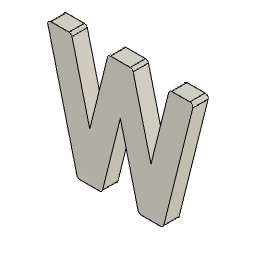
West (Autodesk Fusion 360 design; units mm, degrees)
Autodesk Fusion 360 part; units mm, degrees
sketch "Sketch1" plane through (0, 0, 0) normal (0, 1, 0) x (1, 0, 0)
  line L0 (1.6266, -50.8) -> (9.1684, -50.8)
  line L1 (0.3945, -49.222) -> (12.4595, -0.962)
  line L2 (13.6916, 0) -> (21.8684, 0)
  line L3 (26.3916, -50.8) -> (34.5684, -50.8)
  line L4 (30.48, -30.48) -> (23.1005, -0.962)
  line L5 (30.48, -30.48) -> (37.8595, -0.962)
  line L6 (39.0916, 0) -> (47.2684, 0)
  line L7 (43.18, -20.32) -> (35.8005, -49.838)
  line L8 (43.18, -20.32) -> (50.5595, -49.838)
  line L9 (51.7916, -50.8) -> (59.3334, -50.8)
  line L10 (60.5655, -49.222) -> (48.5005, -0.962)
  arc A0 (0.3945, -49.222) -> (1.6266, -50.8) centre (1.6266, -49.53) ccw
  arc A1 (9.1684, -50.8) -> (10.4005, -49.838) centre (9.1684, -49.53) ccw
  arc A2 (13.6916, 0) -> (12.4595, -0.962) centre (13.6916, -1.27) ccw
  arc A3 (23.1005, -0.962) -> (21.8684, 0) centre (21.8684, -1.27) ccw
  arc A4 (39.0916, 0) -> (37.8595, -0.962) centre (39.0916, -1.27) ccw
  arc A5 (48.5005, -0.962) -> (47.2684, 0) centre (47.2684, -1.27) ccw
  arc A6 (59.3334, -50.8) -> (60.5655, -49.222) centre (59.3334, -49.53) ccw
  arc A7 (50.5595, -49.838) -> (51.7916, -50.8) centre (51.7916, -49.53) ccw
  arc A8 (34.5684, -50.8) -> (35.8005, -49.838) centre (34.5684, -49.53) ccw
  arc A9 (25.1595, -49.838) -> (26.3916, -50.8) centre (26.3916, -49.53) ccw
  line L11 (17.78, -20.32) -> (10.4005, -49.838)
  line L12 (17.78, -20.32) -> (25.1595, -49.838)
  dimension "d1" = 1.27
  constraint horizontal L0
  constraint parallel L0 L2
  constraint parallel L2 L3
  constraint parallel L3 L6
  constraint parallel L5 L7
  constraint parallel L4 L8
  constraint parallel L6 L9
  constraint parallel L8 L10
  constraint tangent L0 A0
  constraint tangent L1 A0
  constraint tangent L0 A1
  constraint equal A0 A1
  constraint tangent L1 A2
  constraint tangent L2 A2
  constraint equal A0 A2
  constraint tangent L2 A3
  constraint tangent L4 A3
  constraint equal A0 A3
  constraint tangent L5 A4
  constraint tangent L6 A4
  constraint equal A0 A4
  constraint tangent L6 A5
  constraint tangent L10 A5
  constraint equal A0 A5
  constraint tangent L9 A6
  constraint tangent L10 A6
  constraint equal A0 A6
  constraint tangent L8 A7
  constraint tangent L9 A7
  constraint equal A0 A7
  constraint tangent L7 A8
  constraint tangent L3 A8
  constraint equal A0 A8
  constraint tangent L3 A9
  constraint equal A0 A9
  measures "d1" radius of A0
extrude "Extrude1" add sketch "Sketch1" along normal blind 6.35
